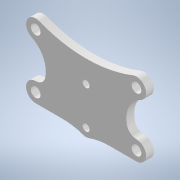
# Autodesk Inventor part: AS5600_mount
Saved by Autodesk Inventor 2022 (Build 260153070, 153G)
## iProperties
Created: 2021-10-29
Part Number: AS5600_mount
Material: Generic
Document SubType Name: Modeling
Designer: a laptop
Density: 1 g/cm^3
Appearance: Default
Author: a laptop
Autodesk Inventor part; units mm, degrees
ref_plane "YZ Plane" through (0, 0, 0) normal (1, 0, 0) x (0, 1, 0)
ref_plane "XZ Plane" through (0, 0, 0) normal (0, 1, 0) x (-1, 0, 0)
ref_plane "XY Plane" through (0, 0, 0) normal (0, 0, 1) x (1, 0, 0)
sketch "Sketch1" plane through (0, 0, 0) normal (0, 0, 1) x (1, 0, 0)
  circle A0 centre (0, -6) radius 1.1 projected
  circle A1 centre (0, 6) radius 1.1 projected
  circle A2 centre (-16, 13) radius 1.55 projected
  circle A3 centre (16, 13) radius 1.55 projected
  circle A4 centre (-16, -4.25) radius 1.55 projected
  circle A5 centre (16, -4.25) radius 1.55 projected
  arc A6 (17.7494, -6.7484) -> (16, -1.2) centre (16, -4.25) ccw projected
  arc A7 (12.9233, 1.4645) -> (16, -1.2) centre (16, 1.9085) ccw projected
  arc A8 (17.3284, 10.2545) -> (12.8667, 1.8571) centre (20.8351, 3.0073) ccw projected
  line L0 (12.9233, 1.4645) -> (12.8667, 1.8571) projected
  arc A9 (17.3284, 10.2545) -> (14.878, 15.8361) centre (16, 13) ccw projected
  arc A10 (-14.878, 15.8361) -> (14.878, 15.8361) centre (0, 53.4422) ccw projected
  arc A11 (-14.878, 15.8361) -> (-17.3284, 10.2545) centre (-16, 13) ccw projected
  arc A12 (-12.8667, 1.8571) -> (-17.3284, 10.2545) centre (-20.8351, 3.0073) ccw projected
  arc A13 (-16, -1.2) -> (-12.9233, 1.4645) centre (-16, 1.9085) ccw projected
  line L1 (-12.8667, 1.8571) -> (-12.9233, 1.4645) projected
  arc A14 (-16, -1.2) -> (-17.7494, -6.7484) centre (-16, -4.25) ccw projected
  line L2 (0, -6) -> (-7.5, -6) construction
  line L3 (-7.5, -6) -> (-7.5, 6) construction
  line L4 (-7.5, 6) -> (0, 6) construction
  line L5 (0, 6) -> (7.5, 6) construction
  line L6 (7.5, 6) -> (7.5, -6) construction
  line L7 (7.5, -6) -> (0, -6) construction
  arc A15 (-17.7494, -6.7484) -> (-16, -7.3) centre (-16, -4.25) ccw
  arc A16 (16, -1.2) -> (16, -7.3) centre (16, -4.25) ccw construction
  line L8 (-16, -7.3) -> (-7.5, -7.3)
  arc A17 (-0.875, -8.4483) -> (0.875, -8.4483) centre (0, -6) ccw
  arc A18 (7.5, -7.3) -> (0.875, -8.4483) centre (7.5, -26.9846) ccw
  arc A19 (-0.875, -8.4483) -> (-7.5, -7.3) centre (-7.5, -26.9846) ccw
  line L9 (-7.5, -7.3) -> (-2.2517, -7.3) construction
  line L10 (7.5, -7.3) -> (16, -7.3)
  arc A20 (-2.2517, -7.3) -> (-0.875, -8.4483) centre (0, -6) ccw construction
  arc A21 (0.875, -8.4483) -> (2.2517, -7.3) centre (0, -6) ccw construction
  arc A22 (2.2517, -7.3) -> (-2.2517, -7.3) centre (0, -6) ccw construction
  line L11 (-2.2517, -7.3) -> (2.2517, -7.3) construction
  line L12 (2.2517, -7.3) -> (7.5, -7.3) construction
  arc A23 (16, -7.3) -> (17.7494, -6.7484) centre (16, -4.25) ccw
  arc A24 (-16, -7.3) -> (-16, -1.2) centre (-16, -4.25) ccw construction
  point P0 (0, 0)
  dimension "d0" = 1.5
  dimension "d1" = 15
  constraints: 25 tangent, 22 end point, 22 point on circle, 10 centre point, 4 perpendicular, 4 point on line, 4 vertical alignment, 1 coincident, 1 collinear, 1 horizontal, 1 parallel
  measures "d0" radial gap between concentric circles of A0 A17
  measures "d1" distance between parallel lines of L6 L3
extrude "Extrusion1" add sketch "Sketch1" along normal blind 2.5
body "Solid1"
